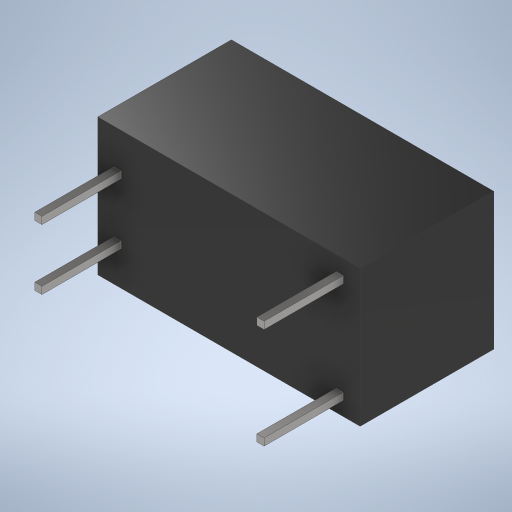
# Autodesk Inventor part: GMS0205
Saved by Autodesk Inventor 2023 (Build 270158000, 158)
## iProperties
Created: 2022-06-23
Part Number: GMS0205
Material: 일반
Document SubType Name: Modeling
Designer: user
Density: 1 g/cm^3
Appearance: 기본값
Author: user
Autodesk Inventor part; units mm, degrees
ref_plane "YZ Plane" through (0, 0, 0) normal (1, 0, 0) x (0, 1, 0)
ref_plane "XZ Plane" through (0, 0, 0) normal (0, 1, 0) x (-1, 0, 0)
ref_plane "XY Plane" through (0, 0, 0) normal (0, 0, 1) x (1, 0, 0)
sketch "스케치1" plane through (0, 0, 0) normal (0, 0, 1) x (1, 0, 0)
  line L0 (-16.5, 8.6) -> (16.5, 8.6)
  line L1 (16.5, 8.6) -> (16.5, -8.6)
  line L2 (16.5, -8.6) -> (-16.5, -8.6)
  line L3 (-16.5, -8.6) -> (-16.5, 8.6)
  line L4 (-16.5, 8.6) -> (16.5, -8.6) construction
  line L5 (16.5, 8.6) -> (-16.5, -8.6) construction
  line L6 (13.52, 6.8) -> (14.42, 6.8)
  line L7 (14.42, 6.8) -> (14.42, 5.9)
  line L8 (14.42, 5.9) -> (13.52, 5.9)
  line L9 (13.52, 5.9) -> (13.52, 6.8)
  line L10 (13.52, 6.8) -> (14.42, 5.9) construction
  line L11 (14.42, 6.8) -> (13.52, 5.9) construction
  line L12 (13.52, -5.9) -> (14.42, -5.9)
  line L13 (14.42, -5.9) -> (14.42, -6.8)
  line L14 (14.42, -6.8) -> (13.52, -6.8)
  line L15 (13.52, -6.8) -> (13.52, -5.9)
  line L16 (13.52, -5.9) -> (14.42, -6.8) construction
  line L17 (14.42, -5.9) -> (13.52, -6.8) construction
  line L18 (-14.42, 3.36) -> (-13.52, 3.36)
  line L19 (-13.52, 3.36) -> (-13.52, 4.26)
  line L20 (-13.52, 4.26) -> (-14.42, 4.26)
  line L21 (-14.42, 4.26) -> (-14.42, 3.36)
  line L22 (-14.42, 3.36) -> (-13.52, 4.26) construction
  line L23 (-13.52, 3.36) -> (-14.42, 4.26) construction
  line L24 (-14.42, -3.36) -> (-13.52, -3.36)
  line L25 (-13.52, -3.36) -> (-13.52, -4.26)
  line L26 (-13.52, -4.26) -> (-14.42, -4.26)
  line L27 (-14.42, -4.26) -> (-14.42, -3.36)
  line L28 (-14.42, -3.36) -> (-13.52, -4.26) construction
  line L29 (-13.52, -3.36) -> (-14.42, -4.26) construction
  point P0 (0, 0)
  point P1 (13.97, 6.35)
  point P2 (13.97, -6.35)
  point P3 (-13.97, 3.81)
  point P4 (-13.97, -3.81)
  dimension "d0" = 33
  dimension "d1" = 17.2
  dimension "d2" = 2.25
  dimension "d3" = 12.7
  dimension "d4" = 0.9
  dimension "d5" = 0.9
  dimension "d6" = 0.9
  dimension "d7" = 0.9
  dimension "d8" = 0.9
  dimension "d9" = 0.9
  dimension "d10" = 0.9
  dimension "d11" = 0.9
  dimension "d12" = 4.79
  dimension "d13" = 7.62
  dimension "d14" = 2.53
  dimension "d15" = 27.94
  constraints: 60 end point, 10 midpoint, 10 parallel, 5 horizontal, 5 perpendicular, 2 vertical alignment
  measures "d0" distance of L1.end L2.end
  measures "d1" distance of L0.end L1.end
  measures "d2" distance from line of L0 point (13.97, 6.35)
  measures "d3" distance of point (13.97, -6.35) point (13.97, 6.35)
  measures "d4" distance of L7.end L8.end
  measures "d5" distance of L8.end L6.start
  measures "d6" distance of L12.start L12.end
  measures "d7" distance of L14.end L12.start
  measures "d8" distance of L20.end L19.end
  measures "d9" distance of L19.end L18.end
  measures "d10" distance of L25.end L26.end
  measures "d11" distance of L24.end L25.end
  measures "d12" distance from line of L0 point (-13.97, 3.81)
  measures "d13" distance of point (-13.97, -3.81) point (-13.97, 3.81)
  measures "d14" distance from line of L3 point (-13.97, -3.81)
  measures "d15" horizontal distance of point (13.97, -6.35) point (-13.97, -3.81)
extrude "돌출1" add sketch "스케치1" against normal blind 16.8 contours L0 L1 L2 L3 | L6 L7 L8 L9 | L12 L13 L14 L15 | L21 L20 L19 L18 | L24 L25 L26 L27
extrude "돌출2" add sketch "스케치1" along normal blind 10 contours L6 L7 L8 L9 | L12 L13 L14 L15 | L21 L20 L19 L18 | L24 L25 L26 L27
